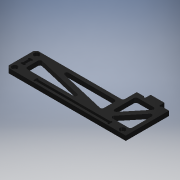
# Autodesk Inventor part: コックピット_2_メインフレーム_2
Saved by Autodesk Inventor 2018 (Build 220112000, 112)
## iProperties
Created: 2016-05-24
Part Number: コックピット_2_メインフレーム_2
Material: アセタール樹脂、黒
Document SubType Name: Modeling
Designer: hiroaki
Density: 1.425 g/cm^3
Appearance: 滑らか - 黒
Mass: 17.2847 g
Surface Area: 94.2011 cm^2
Volume: 12.1296 cm^3
Author: hiroaki
Autodesk Inventor part; units mm, degrees
ref_plane "YZ Plane" through (0, 0, 0) normal (1, 0, 0) x (0, 1, 0)
ref_plane "XZ Plane" through (0, 0, 0) normal (0, 1, 0) x (-1, 0, 0)
ref_plane "XY Plane" through (0, 0, 0) normal (0, 0, 1) x (1, 0, 0)
derived "コックピット_2_基礎_2.ipt"
sketch "スケッチ1" plane through (0, 0, 0) normal (0, 0, 1) x (1, 0, 0)
  line L0 (-63.75, 16) -> (-63.75, -16) construction
  line L1 (-63.75, -16) -> (63.75, -16)
  line L2 (63.75, -16) -> (63.75, 31)
  line L3 (63.75, 31) -> (55.85, 31)
  line L4 (-63.75, 16) -> (28.75, 16)
  line L5 (28.75, 16) -> (28.75, 31)
  line L6 (28.75, 31) -> (36.65, 31)
  line L7 (38.75, 31) -> (38.75, 36)
  line L8 (38.75, 36) -> (53.75, 36)
  line L9 (53.75, 36) -> (53.75, 31)
  arc A0 (36.65, 31) -> (38.75, 31) centre (37.7, 31) ccw
  arc A1 (53.75, 31) -> (55.85, 31) centre (54.8, 31) ccw
  line L10 (46.25, 36) -> (46.25, -16) construction
  line L11 (-63.75, 16) -> (-58.75, 16) construction
  line L12 (-58.75, 16) -> (-58.75, -16) construction
  line L13 (-58.75, -16) -> (-63.75, -16) construction
  line L14 (-63.75, -16) -> (-63.75, 16) construction
  line L15 (-58.75, -16) -> (63.75, -16) construction
  line L16 (63.75, -16) -> (63.75, -11) construction
  line L17 (63.75, -11) -> (-58.75, -11) construction
  line L18 (-58.75, -11) -> (-58.75, -16) construction
  circle A2 centre (-61.25, 12) radius 1.55
  circle A3 centre (-61.25, -12) radius 1.55
  line L19 (-63.75, 0) -> (-58.75, 0) construction
  line L20 (-63.75, 16) -> (-66.25, 13.5)
  line L21 (-66.25, 13.5) -> (-66.25, -13.5)
  line L22 (-66.25, -13.5) -> (-63.75, -16)
  circle A4 centre (-61.25, 12) radius 3 construction
  line L23 (-58.75, 5) -> (-61.25, 5) construction
  line L24 (-61.25, 5) -> (-61.25, -5) construction
  line L25 (-61.25, -5) -> (-58.75, -5) construction
  line L26 (-58.75, -5) -> (-58.75, 5) construction
  line L27 (-38.75, -11) -> (43.75, -11) construction
  line L28 (43.75, -11) -> (43.75, -13.5) construction
  line L29 (43.75, -13.5) -> (-38.75, -13.5) construction
  line L30 (-38.75, -13.5) -> (-38.75, -11) construction
  line L31 (-61.3, -5.05) -> (-61.3, 5.05)
  line L32 (-61.3, 5.05) -> (-58.7, 5.05)
  line L33 (-58.7, 5.05) -> (-58.7, -5.05)
  line L34 (-58.7, -5.05) -> (-61.3, -5.05)
  circle A5 centre (-61.3, -4) radius 1.05
  circle A6 centre (-58.7, -4) radius 1.05
  circle A7 centre (-61.3, 4) radius 1.05
  circle A8 centre (-58.7, 4) radius 1.05
  line L35 (-38.8, -10.95) -> (43.8, -10.95)
  line L36 (43.8, -10.95) -> (43.8, -13.55)
  line L37 (43.8, -13.55) -> (-38.8, -13.55)
  line L38 (-38.8, -13.55) -> (-38.8, -10.95)
  circle A9 centre (-37.75, -13.55) radius 1.05
  circle A10 centre (-37.75, -10.95) radius 1.05
  circle A11 centre (42.75, -10.95) radius 1.05
  circle A12 centre (42.75, -13.55) radius 1.05
  line L39 (-2.5, 52.75) -> (-2.5, -37.25) construction
  circle A13 centre (56.25, -12) radius 1.55
  point P0 (0, 0)
  point P1 (0, -16)
  point P2 (-61.25, 16)
  dimension "d13" = 2.1
  dimension "d14" = 0.05
  dimension "d15" = 0.05
  measures "d14" distance between parallel lines of L31 L24
  measures "d15" distance between parallel lines of L38 L30
extrude "押し出し1" add sketch "スケッチ1" along normal blind 5
sketch "スケッチ3" plane through (28.75, 31, 0) normal (0, 1, 0) x (1, 0, 0)
  line L0 (0, 0) -> (0, -5) projected
  line L1 (35, 0) -> (35, -5) projected
  point P0 (-28.75, 0)
  point P1 (31, -2.5)
  point P2 (4, -2.5)
  point P3 (0, -2.5)
  dimension "d3" = 27
  dimension "d4" = 35
  dimension "d5" = 4
  constraints: 2 horizontal alignment, 1 midpoint
  measures "d3" distance of point (4, -2.5) point (31, -2.5)
  measures "d4" distance between parallel lines of L1 L0
  measures "d5" distance from line of L0 point (4, -2.5)
hole "穴1" at (59.75, 31, 2.5) at (32.75, 31, 2.5) direction (0, -1, 0) diameter 2.459 depth 2.5 thread size "M3x0.5" class "6H" standard "ISO Metric profile"
sketch "スケッチ4" plane through (-63.75, -16, 5) normal (0, 0, 1) x (1, 0, 0)
  line L0 (105.45, 2.45) -> (27.05, 2.45) projected
  arc A0 (24.95, 2.45) -> (27.05, 2.45) centre (26, 2.45) ccw projected
  line L1 (24.95, 2.45) -> (24.95, 5.05) projected
  arc A1 (27.05, 5.05) -> (24.95, 5.05) centre (26, 5.05) ccw projected
  line L2 (27.05, 5.05) -> (105.45, 5.05) projected
  arc A2 (107.55, 5.05) -> (105.45, 5.05) centre (106.5, 5.05) ccw projected
  line L3 (107.55, 5.05) -> (107.55, 2.45) projected
  arc A3 (105.45, 2.45) -> (107.55, 2.45) centre (106.5, 2.45) ccw projected
  line L4 (127.5, 0) -> (127.5, 47) projected
  line L5 (100.4, 47) -> (92.5, 47) projected
  line L6 (92.5, 47) -> (92.5, 32) projected
  line L7 (92.5, 32) -> (0, 32) projected
  line L8 (5.05, 18.95) -> (5.05, 13.05) projected
  arc A4 (5.05, 10.95) -> (5.05, 13.05) centre (5.05, 12) ccw projected
  line L9 (5.05, 10.95) -> (2.45, 10.95) projected
  arc A5 (2.45, 13.05) -> (2.45, 10.95) centre (2.45, 12) ccw projected
  line L10 (2.45, 13.05) -> (2.45, 18.95) projected
  arc A6 (2.45, 21.05) -> (2.45, 18.95) centre (2.45, 20) ccw projected
  line L11 (2.45, 21.05) -> (5.05, 21.05) projected
  arc A7 (5.05, 18.95) -> (5.05, 21.05) centre (5.05, 20) ccw projected
  line L12 (9, 28) -> (89.5, 28) construction
  line L13 (89.5, 28) -> (89.5, 9) construction
  line L14 (89.5, 9) -> (9, 9) construction
  line L15 (9, 9) -> (9, 28) construction
  line L16 (96.5, 42) -> (123.5, 42) construction
  line L17 (123.5, 42) -> (123.5, 9) construction
  line L18 (123.5, 9) -> (96.5, 9) construction
  line L19 (96.5, 9) -> (96.5, 42) construction
  line L20 (9, 28) -> (89.5, 9) construction
  line L21 (96.5, 9) -> (123.5, 42) construction
  line L22 (19.8831, 28) -> (89.5, 28)
  line L23 (89.5, 28) -> (89.5, 11.5687)
  line L24 (89.5, 11.5687) -> (19.8831, 28)
  line L25 (9, 25.4313) -> (9, 9)
  line L26 (9, 9) -> (78.6169, 9)
  line L27 (78.6169, 9) -> (9, 25.4313)
  line L28 (5.05, 21) -> (2.45, 21) construction
  arc A8 (2.45, 21) -> (2.5, 19.0013) centre (2.45, 20) ccw construction
  line L29 (2.5, 19.0013) -> (2.5, 12.9987) construction
  arc A9 (2.5, 12.9987) -> (2.45, 11) centre (2.45, 12) ccw construction
  line L30 (2.45, 11) -> (5.05, 11) construction
  arc A10 (5.05, 11) -> (5, 12.9987) centre (5.05, 12) ccw construction
  line L31 (5, 12.9987) -> (5, 19.0013) construction
  arc A11 (5, 19.0013) -> (5.05, 21) centre (5.05, 20) ccw construction
  line L32 (105.5013, 5) -> (26.9987, 5) construction
  arc A12 (26.9987, 5) -> (25, 5.05) centre (26, 5.05) ccw construction
  line L33 (25, 5.05) -> (25, 2.45) construction
  arc A13 (25, 2.45) -> (26.9987, 2.5) centre (26, 2.45) ccw construction
  line L34 (26.9987, 2.5) -> (105.5013, 2.5) construction
  arc A14 (105.5013, 2.5) -> (107.5, 2.45) centre (106.5, 2.45) ccw construction
  line L35 (107.5, 2.45) -> (107.5, 5.05) construction
  arc A15 (107.5, 5.05) -> (105.5013, 5) centre (106.5, 5.05) ccw construction
  line L36 (96.5, 42) -> (120.2698, 42)
  line L37 (120.2698, 42) -> (96.5, 12.948)
  line L38 (96.5, 12.948) -> (96.5, 42)
  line L39 (99.7302, 9) -> (123.5, 9)
  line L40 (123.5, 9) -> (123.5, 38.052)
  line L41 (123.5, 38.052) -> (99.7302, 9)
  point P0 (63.75, 16)
  dimension "d16" = 0.05
  dimension "d17" = 4
  dimension "d18" = 4
  dimension "d19" = 0.05
  dimension "d20" = 4
  dimension "d21" = 5
  dimension "d22" = 3
  dimension "d23" = 4
  dimension "d24" = 4
  dimension "d25" = 5
  dimension "d26" = 5
  constraints: 60 end point, 16 point on circle, 9 collinear, 8 centre point, 8 parallel, 5 horizontal, 5 perpendicular, 1 point on line, 1 vertical, 16 other
  measures "d16" distance between parallel lines of L8 L31
  measures "d17" distance between parallel lines of L15 L31
  measures "d18" distance between parallel lines of L7 L12
  measures "d19" distance between parallel lines of L2 L32
  measures "d20" distance between parallel lines of L14 L32
  measures "d21" distance between parallel lines of L27 L24
  measures "d22" distance between parallel lines of L6 L13
  measures "d23" distance between parallel lines of L19 L6
  measures "d24" distance between parallel lines of L4 L17
  measures "d25" distance between parallel lines of L16 L5
  measures "d26" distance between parallel lines of L41 L37
extrude "押し出し2" cut sketch "スケッチ4" against normal blind 10 contours L22 L23 L24 | L27 L26 L25 | L36 L37 L38 | L41 L40 L39
fillet "フィレット1" radius 2 13 edges at (-43.8669, 12, 2.5) (14.8669, -7, 2.5) (25.75, -4.4313, 2.5) (32.75, -3.052, 2.5) (35.9802, -7, 2.5) (-54.75, -7, 2.5) (59.75, -7, 2.5) (56.5198, 26, 2.5) (59.75, 22.052, 2.5) (32.75, 26, 2.5) (25.75, 12, 2.5) (-54.75, 9.4313, 2.5) (28.75, 16, 2.5)
sketch "スケッチ5" plane through (-63.75, -16, 5) normal (0, 0, 1) x (1, 0, 0)
  circle A0 centre (2.5, 28) radius 1.55 projected
  circle A1 centre (2.5, 4) radius 1.55 projected
  circle A2 centre (120, 4) radius 1.55 projected
  point P0 (63.75, 16)
  point P1 (2.5, 28)
  point P2 (2.5, 4)
  constraints: 3 coincident
hole "穴2" at (-61.25, 12, 5) at (-61.25, -12, 5) at (56.25, -12, 5) direction (0, 0, -1) diameter 6 depth 3.5
equation "\"d5\" = -0.5 * d3 + 0.5 * d4"
equation "\"d20\" = d17"
equation "\"d23\" = d18"
equation "\"d24\" = d18"
